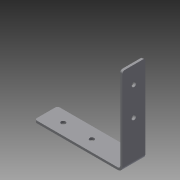
# Autodesk Inventor part: angleBracket
Saved by Autodesk Inventor 2014 (Build 180170000, 170)
## iProperties
Created: 2014-08-29
Part Number: angleBracket
Material: Generic
Document SubType Name: Sheet Metal
Designer: Dave
Density: 1 g/cm^3
Appearance: Default
Sheet Metal Rule: Default
Author: Dave
Autodesk Inventor part; units mm, degrees
ref_plane "YZ Plane" through (0, 0, 0) normal (1, 0, 0) x (0, 1, 0)
ref_plane "XZ Plane" through (0, 0, 0) normal (0, 1, 0) x (-1, 0, 0)
ref_plane "XY Plane" through (0, 0, 0) normal (0, 0, 1) x (1, 0, 0)
sketch "Sketch6" plane through (0, 0, 0) normal (0, 1, 0) x (-1, 0, 0)
  line L0 (0, 0) -> (150, 0)
  line L1 (150, 0) -> (150, 20)
  line L2 (150, 20) -> (0, 20)
  line L3 (0, 20) -> (0, 0)
  dimension "d42" = 150
  dimension "d43" = 20
  constraints: 8 end point, 2 parallel, 1 horizontal, 1 perpendicular
  measures "d42" distance of L0.start L0.end
  measures "d43" distance of L2.end L0.start
extrude "Extrusion3" add sketch "Sketch6" along normal blind 2
fillet "Fillet2" radius 2 4 edges at (-150, 1, 20) (0, 1, 20) (0, 1, 0) (-150, 1, 0)
sketch "Sketch7" plane through (0, 2, 0) normal (0, 1, 0) x (1, 0, 0)
  line L0 (-150, -2) -> (-150, -18) projected
  line L1 (-148, -20) -> (-2, -20) projected
  line L2 (-2, 0) -> (-148, 0) projected
  circle A0 centre (-135, -10) radius 1.3577
  line L3 (-75, 0) -> (-75, -20) construction
  circle A1 centre (-15, -10) radius 1.3577
  line L4 (-150, -10) -> (-75, -10) construction
  point P0 (0, 0)
  dimension "d48" = 60
  constraints: 4 end point, 4 midpoint, 2 centre point, 1 point on line, 1 symmetric about line, 1 other
  measures "d48" distance from line of L3 A0.centre
hole "Hole3" at (-135, 2, 10) at (-15, 2, 10) direction (0, -1, 0) diameter 4 end through all
sketch "Sketch8" plane through (0, 2, 0) normal (0, 1, 0) x (1, 0, 0)
  line L0 (-148, -20) -> (-2, -20) projected
  line L1 (-2, 0) -> (-148, 0) projected
  line L2 (-75, 0) -> (-75, -20)
  point P0 (0, 0)
  constraints: 2 end point, 2 midpoint
fold "Fold1" angle 90 bend radius 2 thickness 2 k factor 0.44 line from (-75, 2, 0) to (-75, 2, 20) line at bend centre moving side (1, 0, 0) folds toward (0, 1, 0)
sketch "Sketch9" plane through (0, 2, 0) normal (0, 1, 0) x (1, 0, 0)
  circle A0 centre (-110, -10) radius 2.3919
  circle A1 centre (-135, -10) radius 2 projected
  point P0 (0, 0)
  dimension "d69" = 25
  constraints: 1 centre point
  measures "d69" distance of A0.centre A1.centre
hole "Hole4" at (-110, 2, 10) direction (0, -1, 0) diameter 4 end through all
sketch "Sketch10" plane through (-75.2619, 4, 20) normal (-1, 0, 0) x (0, 0, 1)
  circle A0 centre (-10, 57.7381) radius 2 projected
  circle A1 centre (-10, 32.7381) radius 1.9296
  point P0 (-20, -4)
  dimension "d70" = 25
  constraints: 1 centre point
  measures "d70" distance of A1.centre A0.centre
hole "Hole5" at (-75.2619, 36.7381, 10) direction (1, 0, 0) diameter 4 end through all
equation "\"d44\" = Thickness"
equation "\"d56\" = BendReliefWidth"
equation "\"d57\" = BendReliefDepth"
equation "\"d58\" = MinimumRemnant"
equation "\"d59\" = BendRadius"
equation "\"d61\" = BendRadius"
equation "\"BendRadius\" = Thickness"
equation "\"BendReliefWidth\" = Thickness"
equation "\"BendReliefDepth\" = 0.5 * Thickness"
equation "\"CornerReliefSize\" = 4 * Thickness"
equation "\"MinimumRemnant\" = 2 * Thickness"
equation "\"TransitionRadius\" = BendRadius"
equation "\"JacobiRadiusSize\" = Thickness"
equation "\"GapSize\" = Thickness"
equation "\"Thickness\" = 2"
body "Solid2"
